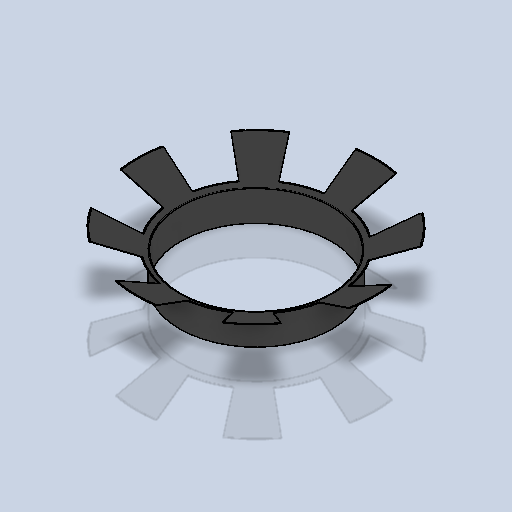
# Autodesk Inventor part: rubber_sleeve
Saved by Autodesk Inventor 2026.1 (Build 301233000, 233)
## iProperties
Created: 2025-09-05
Part Number: rubber_sleeve
Material: Rubber
Document SubType Name: Modeling
Designer: baseb
Density: 0.93 g/cm^3
Appearance: Rubber - Black
Author: baseb
Autodesk Inventor part; units mm, degrees
ref_plane "YZ Plane" through (0, 0, 0) normal (1, 0, 0) x (0, 1, 0)
ref_plane "XZ Plane" through (0, 0, 0) normal (0, 1, 0) x (-1, 0, 0)
ref_plane "XY Plane" through (0, 0, 0) normal (0, 0, 1) x (1, 0, 0)
sketch "Sketch1" plane through (0, 0, 0) normal (1, 0, 0) x (0, 1, 0)
  line L0 (-22.225, 0.762) -> (22.225, 0.762)
  line L1 (22.225, -0.762) -> (-22.225, -0.762)
  line L2 (-22.225, -0.762) -> (-22.225, 0.762)
  line L3 (-22.225, 0.762) -> (22.225, -0.762) construction
  line L4 (22.225, 0.762) -> (-22.225, -0.762) construction
  line L5 (22.225, 0.762) -> (51.435, 64.262)
  line L6 (51.435, 64.262) -> (51.435, 62.738)
  line L7 (51.435, 62.738) -> (22.225, -0.762)
  line L8 (0, -0.762) -> (0, -111.887)
  line L9 (0, -111.887) -> (16.3991, -111.887)
  point P0 (0, 0)
  dimension "d1" = 44.45
  dimension "d2" = 63.5
  dimension "d5" = 1.524
  dimension "d6" = 111.125
  dimension "d8" = 29.21
  dimension "d9" = 1.524
  constraints: 20 end point, 3 midpoint, 2 horizontal, 2 vertical, 1 parallel
  measures "d1" distance of L1.start L1.end
  measures "d2" distance from line of L5.end L0
  measures "d5" distance of L5.end L6.end
  measures "d6" distance of L8.start L8.end
  measures "d8" horizontal distance of L1.start L5.end
  measures "d9" distance of L1.end L0.start
revolve "Revolution1" add sketch "Sketch1" angle 360 about axis through (0, 0, -111.887) along (0, 1, 0)
sketch "Sketch2" plane through (0, 51.435, -111.887) normal (0, 1, 0) x (1, 0, 0)
  circle A0 centre (0, 0) radius 111.125 projected
  circle A1 centre (0, 0) radius 176.149 projected
  line L0 (26.2346, -174.1844) -> (-24.5654, -174.1844) construction
  arc A2 (26.2346, -174.1844) -> (97.3464, -146.8065) centre (0, 0) ccw
  line L1 (0, 0) -> (26.2346, -174.1844) construction
  line L2 (0, 0) -> (97.3464, -146.8065) construction
  arc A3 (16.5503, -109.8856) -> (61.4117, -92.6141) centre (0, 0) ccw
  line L3 (16.5503, -109.8856) -> (26.2346, -174.1844)
  line L4 (97.3464, -146.8065) -> (61.4117, -92.6141)
  dimension "d19" = 50.8
  dimension "d20" = 76.2
  constraints: 10 end point, 8 point on circle, 2 centre point, 2 concentric, 2 point on line
  measures "d19" distance of L0.start L0.end
  measures "d20" distance of L0.start L2.end
extrude "Extrusion2" cut sketch "Sketch2" against normal blind 25.4 contours A0 L4 A1 L3 picked at (28.0302, -151.7692)
pattern_circular "Circular Pattern2" count 8 over 360 about axis through (0, 36.83, -111.887) along (0, 1, 0) of "Extrusion2"
body "Solid1"
